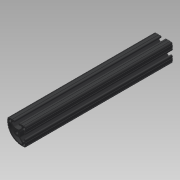
# Autodesk Inventor part: 1517
Saved by Autodesk Inventor 2013 (Build 170138000, 138)
## iProperties
Company: 80/20 Inc.
Created: 2014-04-23
Part Number: 1517
Material: Generic
Document SubType Name: Modeling
Density: 1 g/cm^3
Vendor: 80/20 Inc.
Engineer: Ross Bowman
Designer: Ross Bowman
Catalog Web Link: 8020.net
Material: 6105-T5 Aluminum
Author: Ross Bowman
Keywords: 80/20 , 8020 , T-Slot , Extrusion
Autodesk Inventor part; units mm, degrees
ref_plane "YZ Plane" through (0, 0, 0) normal (1, 0, 0) x (0, 1, 0)
ref_plane "XZ Plane" through (0, 0, 0) normal (0, 1, 0) x (-1, 0, 0)
ref_plane "XY Plane" through (0, 0, 0) normal (0, 0, 1) x (1, 0, 0)
sketch "Sketch1" plane through (0, 0, 0) normal (0, 0, 1) x (1, 0, 0)
  arc A0 (-17.272, 12.1412) -> (-17.018, 11.8872) centre (-17.018, 12.1412) ccw
  line L0 (-17.272, 15.0876) -> (-17.272, 12.1412)
  arc A1 (-15.1384, 17.2212) -> (-17.272, 15.0876) centre (-15.1384, 15.0876) ccw
  line L1 (-12.1412, 17.2212) -> (-15.1384, 17.2212)
  arc A2 (-11.8872, 16.9672) -> (-12.1412, 17.2212) centre (-12.1412, 16.9672) ccw
  line L2 (-11.8872, 12.1412) -> (-11.8872, 16.9672)
  arc A3 (-12.1412, 11.8872) -> (-11.8872, 12.1412) centre (-12.1412, 12.1412) ccw
  line L3 (-17.018, 11.8872) -> (-12.1412, 11.8872)
  circle A4 centre (0, 0) radius 3.3274
  arc A5 (9.269, -16.0372) -> (10.5713, -14.7676) centre (9.3013, -14.7676) ccw
  arc A6 (-16.0341, 9.2879) -> (9.269, -16.0372) centre (9.4921, 9.4888) ccw
  arc A7 (-14.7642, 10.5679) -> (-16.0341, 9.2879) centre (-14.7642, 9.2979) ccw
  line L4 (-12.9549, 10.5679) -> (-14.7642, 10.5679)
  arc A8 (-12.3263, 10.3075) -> (-12.9549, 10.5679) centre (-12.9549, 9.6789) ccw
  line L5 (-7.1284, 5.1096) -> (-12.3263, 10.3075)
  arc A9 (-6.7564, 4.2116) -> (-7.1284, 5.1096) centre (-8.0264, 4.2116) ccw
  line L6 (-6.7564, 0) -> (-6.7564, 4.2116)
  arc A10 (-6.7564, 0) -> (0, -6.7564) centre (0, 0) ccw
  line L7 (3.9386, -6.7564) -> (0, -6.7564)
  arc A11 (4.8366, -7.1284) -> (3.9386, -6.7564) centre (3.9386, -8.0264) ccw
  line L8 (10.311, -12.6027) -> (4.8366, -7.1284)
  arc A12 (10.5713, -13.2314) -> (10.311, -12.6027) centre (9.6823, -13.2314) ccw
  line L9 (10.5713, -14.7676) -> (10.5713, -13.2314)
  arc A13 (12.1463, -11.8401) -> (11.8923, -12.0941) centre (12.1463, -12.0941) ccw
  line L10 (17.018, -11.8401) -> (12.1463, -11.8401)
  arc A14 (17.272, -12.0941) -> (17.018, -11.8401) centre (17.018, -12.0941) ccw
  line L11 (17.272, -15.0876) -> (17.272, -12.0941)
  arc A15 (15.1384, -17.2212) -> (17.272, -15.0876) centre (15.1384, -15.0876) ccw
  line L12 (12.1463, -17.2212) -> (15.1384, -17.2212)
  arc A16 (11.8923, -16.9672) -> (12.1463, -17.2212) centre (12.1463, -16.9672) ccw
  line L13 (11.8923, -12.0941) -> (11.8923, -16.9672)
  arc A17 (12.1412, 17.2212) -> (11.8872, 16.9672) centre (12.1412, 16.9672) ccw
  line L14 (15.1384, 17.2212) -> (12.1412, 17.2212)
  arc A18 (17.272, 15.0876) -> (15.1384, 17.2212) centre (15.1384, 15.0876) ccw
  line L15 (17.272, 12.0941) -> (17.272, 15.0876)
  arc A19 (17.018, 11.8401) -> (17.272, 12.0941) centre (17.018, 12.0941) ccw
  line L16 (12.1412, 11.8401) -> (17.018, 11.8401)
  arc A20 (11.8872, 12.0941) -> (12.1412, 11.8401) centre (12.1412, 12.0941) ccw
  line L17 (11.8872, 16.9672) -> (11.8872, 12.0941)
  arc A21 (-5.8558, 8.1476) -> (-2.4972, 6.7564) centre (-2.4972, 11.5062) ccw
  line L18 (-5.8558, 8.1476) -> (-10.1754, 12.4672)
  arc A22 (-10.287, 12.7366) -> (-10.1754, 12.4672) centre (-9.906, 12.7366) ccw
  line L19 (-10.287, 12.7366) -> (-10.287, 14.5699)
  arc A23 (-8.8932, 15.9637) -> (-10.287, 14.5699) centre (-8.8932, 14.5699) ccw
  line L20 (-8.8932, 15.9637) -> (-6.9992, 15.9637)
  arc A24 (-6.6182, 15.5827) -> (-6.9992, 15.9637) centre (-6.9992, 15.5827) ccw
  line L21 (-6.6182, 15.5827) -> (-6.6182, 15.367)
  arc A25 (-6.6182, 15.367) -> (-6.2372, 14.986) centre (-6.2372, 15.367) ccw
  line L22 (-6.2372, 14.986) -> (-5.6388, 14.986)
  arc A26 (-5.6388, 14.986) -> (-4.064, 16.5608) centre (-5.6388, 16.5608) ccw
  line L23 (-4.064, 16.5608) -> (-4.064, 17.4752)
  arc A27 (-4.064, 17.4752) -> (-5.6388, 19.05) centre (-5.6388, 17.4752) ccw
  line L24 (-5.6388, 19.05) -> (-7.9758, 19.05)
  arc A28 (-9.4998, 19.05) -> (-7.9758, 19.05) centre (-8.7378, 19.05) ccw
  line L25 (-9.4998, 19.05) -> (-14.3282, 19.05)
  arc A29 (-15.8522, 19.05) -> (-14.3282, 19.05) centre (-15.0902, 19.05) ccw
  line L26 (-15.8522, 19.05) -> (-15.8759, 19.05)
  arc A30 (-15.8759, 19.05) -> (-19.0509, 15.8761) centre (-15.8759, 15.875) ccw
  line L27 (-19.0509, 15.8761) -> (-19.0508, 15.8506)
  arc A31 (-19.05, 14.3266) -> (-19.0508, 15.8506) centre (-19.0504, 15.0886) ccw
  line L28 (-19.05, 14.3266) -> (-19.05, 9.525)
  arc A32 (-19.05, 9.525) -> (-18.2241, 2.6723) centre (9.4921, 9.4888) ccw
  arc A33 (-17.8208, 1.2027) -> (-18.2241, 2.6723) centre (-18.0323, 1.9348) ccw
  arc A34 (-17.8208, 1.2027) -> (-16.0569, -3.0251) centre (9.3479, 10.0565) ccw
  arc A35 (-15.3417, -4.3707) -> (-16.0569, -3.0251) centre (-15.7082, -3.7026) ccw
  arc A36 (-15.3417, -4.3707) -> (-10.5738, -10.4703) centre (9.348, 10.0152) ccw
  arc A37 (-10.5738, -10.4703) -> (-4.4477, -15.1275) centre (9.6252, 9.7419) ccw
  arc A38 (-3.1021, -15.8427) -> (-4.4477, -15.1275) centre (-3.7797, -15.4941) ccw
  arc A39 (-3.1021, -15.8427) -> (1.3376, -17.6058) centre (9.6276, 9.7402) ccw
  arc A40 (2.8072, -18.0091) -> (1.3376, -17.6058) centre (2.0697, -17.8173) ccw
  arc A41 (2.8072, -18.0091) -> (9.5111, -19.05) centre (10.5124, 9.5075) ccw
  line L29 (9.5111, -19.05) -> (14.3136, -19.05)
  arc A42 (15.8376, -19.0507) -> (14.3136, -19.05) centre (15.0756, -19.0504) ccw
  arc A43 (15.8376, -19.0507) -> (19.05, -15.7367) centre (15.8781, -15.876) ccw
  arc A44 (19.05, -14.2127) -> (19.05, -15.7367) centre (19.05, -14.9747) ccw
  line L30 (19.05, -14.2127) -> (19.05, -9.4945)
  arc A45 (19.05, -7.9705) -> (19.05, -9.4945) centre (19.05, -8.7325) ccw
  line L31 (19.05, -7.9705) -> (19.05, -5.6388)
  arc A46 (19.05, -5.6388) -> (17.4752, -4.064) centre (17.4752, -5.6388) ccw
  line L32 (17.4752, -4.064) -> (16.5608, -4.064)
  arc A47 (16.5608, -4.064) -> (14.986, -5.6388) centre (16.5608, -5.6388) ccw
  line L33 (14.986, -5.6388) -> (14.986, -6.3233)
  arc A48 (14.986, -6.3233) -> (15.367, -6.7043) centre (15.367, -6.3233) ccw
  line L34 (15.367, -6.7043) -> (15.4588, -6.7043)
  arc A49 (15.8398, -7.0853) -> (15.4588, -6.7043) centre (15.4588, -7.0853) ccw
  line L35 (15.8398, -7.0853) -> (15.8398, -9.017)
  arc A50 (14.5698, -10.287) -> (15.8398, -9.017) centre (14.5698, -9.017) ccw
  line L36 (14.5698, -10.287) -> (12.4636, -10.287)
  arc A51 (12.1942, -10.1754) -> (12.4636, -10.287) centre (12.4636, -9.906) ccw
  line L37 (12.1942, -10.1754) -> (8.1486, -6.1298)
  arc A52 (6.7564, -2.7688) -> (8.1486, -6.1298) centre (11.5096, -2.7688) ccw
  line L38 (6.7564, -2.7688) -> (6.7564, 2.7688)
  arc A53 (8.1486, 6.1298) -> (6.7564, 2.7688) centre (11.5096, 2.7688) ccw
  line L39 (8.1486, 6.1298) -> (12.1942, 10.1754)
  arc A54 (12.4636, 10.287) -> (12.1942, 10.1754) centre (12.4636, 9.906) ccw
  line L40 (12.4636, 10.287) -> (14.5036, 10.287)
  arc A55 (15.7736, 9.017) -> (14.5036, 10.287) centre (14.5036, 9.017) ccw
  line L41 (15.7736, 9.017) -> (15.7736, 7.0853)
  arc A56 (15.3926, 6.7043) -> (15.7736, 7.0853) centre (15.3926, 7.0853) ccw
  line L42 (15.3926, 6.7043) -> (15.367, 6.7043)
  arc A57 (15.367, 6.7043) -> (14.986, 6.3233) centre (15.367, 6.3233) ccw
  line L43 (14.986, 6.3233) -> (14.986, 5.6388)
  arc A58 (14.986, 5.6388) -> (16.5608, 4.064) centre (16.5608, 5.6388) ccw
  line L44 (16.5608, 4.064) -> (17.4752, 4.064)
  arc A59 (17.4752, 4.064) -> (19.05, 5.6388) centre (17.4752, 5.6388) ccw
  line L45 (19.05, 5.6388) -> (19.05, 7.9759)
  arc A60 (19.05, 9.4999) -> (19.05, 7.9759) centre (19.05, 8.7379) ccw
  line L46 (19.05, 9.4999) -> (19.05, 14.3284)
  arc A61 (19.05, 15.8524) -> (19.05, 14.3284) centre (19.05, 15.0904) ccw
  line L47 (19.05, 15.8524) -> (19.05, 15.875)
  arc A62 (19.05, 15.875) -> (15.875, 19.05) centre (15.875, 15.875) ccw
  line L48 (15.875, 19.05) -> (15.847, 19.05)
  arc A63 (14.323, 19.05) -> (15.847, 19.05) centre (15.085, 19.05) ccw
  line L49 (14.323, 19.05) -> (9.4946, 19.05)
  arc A64 (7.9706, 19.05) -> (9.4946, 19.05) centre (8.7326, 19.05) ccw
  line L50 (7.9706, 19.05) -> (5.6388, 19.05)
  arc A65 (5.6388, 19.05) -> (4.064, 17.4752) centre (5.6388, 17.4752) ccw
  line L51 (4.064, 17.4752) -> (4.064, 16.5608)
  arc A66 (4.064, 16.5608) -> (5.6388, 14.986) centre (5.6388, 16.5608) ccw
  line L52 (5.6388, 14.986) -> (6.2372, 14.986)
  arc A67 (6.2372, 14.986) -> (6.6182, 15.367) centre (6.2372, 15.367) ccw
  line L53 (6.6182, 15.367) -> (6.6182, 15.5827)
  arc A68 (6.9992, 15.9637) -> (6.6182, 15.5827) centre (6.9992, 15.5827) ccw
  line L54 (6.9992, 15.9637) -> (8.8932, 15.9637)
  arc A69 (10.287, 14.5699) -> (8.8932, 15.9637) centre (8.8932, 14.5699) ccw
  line L55 (10.287, 14.5699) -> (10.287, 12.7366)
  arc A70 (10.1754, 12.4672) -> (10.287, 12.7366) centre (9.906, 12.7366) ccw
  line L56 (10.1754, 12.4672) -> (5.8558, 8.1476)
  arc A71 (2.4972, 6.7564) -> (5.8558, 8.1476) centre (2.4972, 11.5062) ccw
  line L57 (2.4972, 6.7564) -> (-2.4972, 6.7564)
  constraints: 142 point on circle, 116 end point, 72 centre point
extrude "Extrusion1" add sketch "Sketch1" against normal blind 304.8
body "Solid1"
